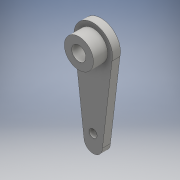
# Autodesk Inventor part: big_servo_arm
Saved by Autodesk Inventor 2016 (Build 200138000, 138)
## iProperties
Created: 2016-04-18
Part Number: big_servo_arm
Material: Generic
Document SubType Name: Modeling
Designer: amenoni
Density: 1 g/cm^3
Appearance: Default
Author: amenoni
Autodesk Inventor part; units mm, degrees
ref_plane "YZ Plane" through (0, 0, 0) normal (1, 0, 0) x (0, 1, 0)
ref_plane "XZ Plane" through (0, 0, 0) normal (0, 1, 0) x (-1, 0, 0)
ref_plane "XY Plane" through (0, 0, 0) normal (0, 0, 1) x (1, 0, 0)
sketch "Sketch1" plane through (0, 0, 0) normal (0, 1, 0) x (-1, 0, 0)
  circle A0 centre (0, 0) radius 2.7
  circle A1 centre (0, 0) radius 5.5
  dimension "d0" = 5.4
  dimension "d1" = 11
  constraints: 2 centre point, 2 coincident
  measures "d0" diameter of A0
  measures "d1" diameter of A1
extrude "Extrusion1" add sketch "Sketch1" along normal blind 5.4
sketch "Sketch2" plane through (0, 5.4, 0) normal (0, 1, 0) x (1, 0, 0)
  circle A0 centre (0, 0) radius 7.3
  dimension "d4" = 14.6
  constraints: 1 centre point, 1 coincident
  measures "d4" diameter of A0
extrude "Extrusion2" add sketch "Sketch2" along normal blind 3
sketch "Sketch3" plane through (0, 8.4, 0) normal (0, 1, 0) x (1, 0, 0)
  arc A0 (3.5, 32) -> (-3.5, 32) centre (0, 32) ccw
  circle A1 centre (0, 0) radius 7.3 projected
  line L0 (-7.3, 0) -> (-3.5, 32)
  line L1 (7.3, 0) -> (3.5, 32)
  dimension "d7" = 7
  dimension "d8" = 32
  constraints: 4 end point, 4 point on circle, 1 centre point
  measures "d7" diameter of A0
  measures "d8" distance of point (0, 0) A0.centre
extrude "Extrusion3" add sketch "Sketch3" against normal blind 3 contours L1 A1 L0 A0 | L1 A1 L0
sketch "Sketch5" plane through (0, 8.4, 0) normal (0, 1, 0) x (1, 0, 0)
  point P0 (0, 0)
  point P1 (0, 28.89)
  dimension "d18" = 28.89
  measures "d18" distance of point (0, 28.89) point (0, 0)
hole "Hole2" at (0, 8.4, -28.89) direction (0, -1, 0) diameter 3 end through all
body "Solid1"
